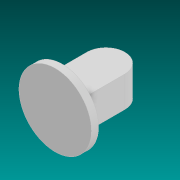
# Autodesk Inventor part: bevestiging axis 2
Saved by Autodesk Inventor 2020.2 (Build 242310000, 310)
## iProperties
Created: 2020-05-18
Part Number: bevestiging axis 2
Material: Generic
Document SubType Name: Modeling
Designer: Svend
Density: 1 g/cm^3
Appearance: Default
Author: Svend
Autodesk Inventor part; units mm, degrees
ref_plane "YZ Plane" through (0, 0, 0) normal (1, 0, 0) x (0, 1, 0)
ref_plane "XZ Plane" through (0, 0, 0) normal (0, 1, 0) x (-1, 0, 0)
ref_plane "XY Plane" through (0, 0, 0) normal (0, 0, 1) x (1, 0, 0)
sketch "Sketch1" plane through (0, 0, 0) normal (0, 0, 1) x (1, 0, 0)
  circle A0 centre (0, 0) radius 50
  dimension "d0" = 100
  constraints: 1 centre point, 1 coincident
  measures "d0" diameter of A0
extrude "Extrusion1" add sketch "Sketch1" along normal blind 10
sketch "Sketch2" plane through (0, 0, 0) normal (0, 1, 0) x (-1, 0, 0)
  circle A0 centre (0, -60) radius 21
  line L0 (50, 0) -> (-50, 0) projected
  circle A1 centre (0, -60) radius 26.1725
  line L1 (-26.1725, -60) -> (-26.1725, 0)
  line L2 (26.1725, -60) -> (26.1725, 0)
  point P0 (0, 0)
  dimension "d3" = 42
  dimension "d10" = 5.1725
  constraints: 4 end point, 2 centre point, 2 perpendicular, 2 point on circle, 2 point on line, 1 vertical alignment
  measures "d3" diameter of A0
  measures "d10" radial gap between concentric circles of A0 A1
extrude "Extrusion3" add sketch "Sketch2" along normal mid plane 42.5 contours A0 | L2 A1 L1 L0 | A1
body "Solid1"
